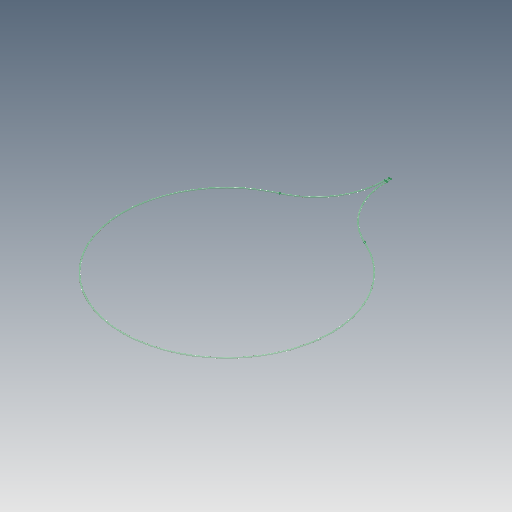
# Autodesk Inventor part: Fiber Loop
Saved by Autodesk Inventor 2020 (Build 240168000, 168)
## iProperties
Created: 2015-08-17
Part Number: Fiber Loop
Material: Glass
Document SubType Name: Modeling
Designer: Cosmic
Density: 2.18 g/cm^3
Appearance: Clear - Green 1
Author: Cosmic
Autodesk Inventor part; units mm, degrees
note: some values were not read from the file. Left out: dimensions or parameters whose unit could not be read.
ref_plane "YZ Plane" through (0, 0, 0) normal (1, 0, 0) x (0, 1, 0)
ref_plane "XZ Plane" through (0, 0, 0) normal (0, 1, 0) x (-1, 0, 0)
ref_plane "XY Plane" through (0, 0, 0) normal (0, 0, 1) x (1, 0, 0)
sketch "Sketch1" plane through (0, 0, 0) normal (0, 0, 1) x (1, 0, 0)
  arc A0 (30.463183, 68.534623) -> (-30.463183, 68.534623) centre (0, 0) ccw
  arc A1 (-30.528171, 68.68083) -> (-33.355077, 67.353281) centre (0, 0) ccw
  arc A2 (-37.826681, 66.079057) -> (-38.359263, 65.77132) centre (0, 0) ccw
  arc A3 (-38.420862, 65.920614) -> (-38.91605, 65.629498) centre (0, 0) ccw
  arc A4 (-1.3, 115.412304) -> (-101.3, 115.412304) centre (-51.3, 115.412304) ccw
  arc A5 (-1.14, 115.412304) -> (-101.46, 115.412304) centre (-51.3, 115.412304) ccw
  arc A6 (-30.528171, 68.68083) -> (-23.706504, 72.355382) centre (-51.3, 115.412304) ccw
  arc A7 (-33.355077, 67.353281) -> (-30.463183, 68.534623) centre (-51.3, 115.412304) ccw
  arc A8 (30.991211, 69.722556) -> (101.3, 115.412304) centre (51.3, 115.412304) ccw
  arc A9 (28.122774, 70.92813) -> (30.926223, 69.576349) centre (51.3, 115.412304) ccw
  arc A10 (23.190762, 72.690292) -> (23.706504, 72.355382) centre (51.3, 115.412304) ccw
  arc A11 (22.642863, 72.862822) -> (23.121211, 72.544532) centre (51.3, 115.412304) ccw
  line L0 (-51.3, 115.412304) -> (51.3, 115.412304)
  arc A12 (-33.808111, 68.401035) -> (-38.420862, 65.920614) centre (0, 0) ccw
  arc A13 (-30.926223, 69.576349) -> (-37.826681, 66.079057) centre (0, 0) ccw
  arc A14 (-37.826681, 66.079057) -> (-30.528171, 68.68083) centre (-51.3, 115.412304) ccw
  arc A15 (-38.359263, 65.77132) -> (-33.355077, 67.353281) centre (-51.3, 115.412304) ccw
  arc A16 (-38.420862, 65.920614) -> (-37.826681, 66.079057) centre (-51.3, 115.412304) ccw
  arc A17 (-38.359263, 65.77132) -> (38.359263, 65.77132) centre (0, 0) ccw
  arc A18 (-0.16, 115.412304) -> (-102.44, 115.412304) centre (-51.3, 115.412304) ccw
  arc A19 (-38.91605, 65.629498) -> (38.91605, 65.629498) centre (0, 0) ccw
  arc A20 (38.359263, 65.77132) -> (37.826681, 66.079057) centre (0, 0) ccw
  arc A21 (38.91605, 65.629498) -> (38.420862, 65.920614) centre (0, 0) ccw
  arc A22 (-102.44, 115.412304) -> (-38.420862, 65.920614) centre (-51.3, 115.412304) ccw
  arc A23 (-38.91605, 65.629498) -> (-38.359263, 65.77132) centre (-51.3, 115.412304) ccw
  arc A24 (0, 115.412304) -> (-102.6, 115.412304) centre (-51.3, 115.412304) ccw
  arc A25 (-23.706504, 72.355382) -> (-23.190762, 72.690292) centre (-51.3, 115.412304) ccw
  arc A26 (-23.190762, 72.690292) -> (-28.122774, 70.92813) centre (0, 0) ccw
  arc A27 (-23.190762, 72.690292) -> (-0.16, 115.412304) centre (-51.3, 115.412304) ccw
  arc A28 (-30.991211, 69.722556) -> (-1.3, 115.412304) centre (-51.3, 115.412304) ccw
  arc A29 (-28.122774, 70.92813) -> (-1.14, 115.412304) centre (-51.3, 115.412304) ccw
  arc A30 (-22.642863, 72.862822) -> (0, 115.412304) centre (-51.3, 115.412304) ccw
  arc A31 (-27.648555, 69.889792) -> (-30.528171, 68.68083) centre (0, 0) ccw
  arc A32 (-30.463183, 68.534623) -> (30.463183, 68.534623) centre (0, 0) ccw
  arc A33 (-33.808111, 68.401035) -> (-30.926223, 69.576349) centre (-51.3, 115.412304) ccw
  arc A34 (-101.46, 115.412304) -> (-33.808111, 68.401035) centre (-51.3, 115.412304) ccw
  arc A35 (-33.355077, 67.353281) -> (33.355077, 67.353281) centre (0, 0) ccw
  arc A36 (-101.3, 115.412304) -> (-30.991211, 69.722556) centre (-51.3, 115.412304) ccw
  arc A37 (-102.6, 115.412304) -> (-38.91605, 65.629498) centre (-51.3, 115.412304) ccw
  arc A38 (33.355077, 67.353281) -> (30.528171, 68.68083) centre (0, 0) ccw
  arc A39 (-30.991211, 69.722556) -> (-33.808111, 68.401035) centre (0, 0) ccw
  arc A40 (-30.926223, 69.576349) -> (-28.122774, 70.92813) centre (-51.3, 115.412304) ccw
  arc A41 (-30.463183, 68.534623) -> (-27.648555, 69.889792) centre (-51.3, 115.412304) ccw
  arc A42 (-27.648555, 69.889792) -> (-23.121211, 72.544532) centre (-51.3, 115.412304) ccw
  arc A43 (-28.122774, 70.92813) -> (-30.991211, 69.722556) centre (0, 0) ccw
  arc A44 (-23.706504, 72.355382) -> (-30.926223, 69.576349) centre (0, 0) ccw
  arc A45 (27.648555, 69.889792) -> (-27.648555, 69.889792) centre (0, 0) ccw
  arc A46 (-23.121211, 72.544532) -> (-22.642863, 72.862822) centre (-51.3, 115.412304) ccw
  arc A47 (-22.642863, 72.862822) -> (-23.190762, 72.690292) centre (0, 0) ccw
  arc A48 (22.642863, 72.862822) -> (-22.642863, 72.862822) centre (0, 0) ccw
  arc A49 (-23.121211, 72.544532) -> (-23.706504, 72.355382) centre (0, 0) ccw
  arc A50 (23.121211, 72.544532) -> (-23.121211, 72.544532) centre (0, 0) ccw
  arc A51 (1.14, 115.412304) -> (28.122774, 70.92813) centre (51.3, 115.412304) ccw
  arc A52 (1.3, 115.412304) -> (30.991211, 69.722556) centre (51.3, 115.412304) ccw
  arc A53 (0, 115.412304) -> (22.642863, 72.862822) centre (51.3, 115.412304) ccw
  arc A54 (0.16, 115.412304) -> (23.190762, 72.690292) centre (51.3, 115.412304) ccw
  arc A55 (23.121211, 72.544532) -> (27.648555, 69.889792) centre (51.3, 115.412304) ccw
  arc A56 (23.190762, 72.690292) -> (22.642863, 72.862822) centre (0, 0) ccw
  arc A57 (23.706504, 72.355382) -> (30.528171, 68.68083) centre (51.3, 115.412304) ccw
  arc A58 (27.648555, 69.889792) -> (30.463183, 68.534623) centre (51.3, 115.412304) ccw
  arc A59 (28.122774, 70.92813) -> (23.190762, 72.690292) centre (0, 0) ccw
  arc A60 (30.528171, 68.68083) -> (37.826681, 66.079057) centre (51.3, 115.412304) ccw
  arc A61 (23.706504, 72.355382) -> (23.121211, 72.544532) centre (0, 0) ccw
  arc A62 (30.926223, 69.576349) -> (23.706504, 72.355382) centre (0, 0) ccw
  arc A63 (30.926223, 69.576349) -> (33.808111, 68.401035) centre (51.3, 115.412304) ccw
  arc A64 (30.991211, 69.722556) -> (28.122774, 70.92813) centre (0, 0) ccw
  arc A65 (30.463183, 68.534623) -> (33.355077, 67.353281) centre (51.3, 115.412304) ccw
  arc A66 (30.528171, 68.68083) -> (27.648555, 69.889792) centre (0, 0) ccw
  arc A67 (33.355077, 67.353281) -> (38.359263, 65.77132) centre (51.3, 115.412304) ccw
  arc A68 (37.826681, 66.079057) -> (38.420862, 65.920614) centre (51.3, 115.412304) ccw
  arc A69 (101.3, 115.412304) -> (1.3, 115.412304) centre (51.3, 115.412304) ccw
  arc A70 (33.808111, 68.401035) -> (101.46, 115.412304) centre (51.3, 115.412304) ccw
  arc A71 (37.826681, 66.079057) -> (30.926223, 69.576349) centre (0, 0) ccw
  arc A72 (33.808111, 68.401035) -> (30.991211, 69.722556) centre (0, 0) ccw
  arc A73 (38.420862, 65.920614) -> (33.808111, 68.401035) centre (0, 0) ccw
  arc A74 (101.46, 115.412304) -> (1.14, 115.412304) centre (51.3, 115.412304) ccw
  arc A75 (38.359263, 65.77132) -> (38.91605, 65.629498) centre (51.3, 115.412304) ccw
  arc A76 (38.91605, 65.629498) -> (102.6, 115.412304) centre (51.3, 115.412304) ccw
  arc A77 (38.420862, 65.920614) -> (102.44, 115.412304) centre (51.3, 115.412304) ccw
  arc A78 (102.44, 115.412304) -> (0.16, 115.412304) centre (51.3, 115.412304) ccw
  arc A79 (102.6, 115.412304) -> (0, 115.412304) centre (51.3, 115.412304) ccw
  dimension "d16" = 0.16
  dimension "d17" = 0.98
  dimension "d18" = 0.16
  dimension "d19" = 150
  dimension "d20" = 0.16
  dimension "d21" = 0.98
  dimension "d22" = 0.16
  dimension "d23" = 100
  dimension "d28" = 0.16
  dimension "d29" = 0.98
  dimension "d30" = 0.16
  dimension "d31" = 100
  constraints: 181 point on circle, 80 centre point, 10 coincident, 3 tangent, 19 other
  measures "d16" radial gap between concentric circles of A1 A0
  measures "d17" radial gap between concentric circles of A2 A1
  measures "d18" radial gap between concentric circles of A3 A2
  measures "d19" diameter of A0
  measures "d20" radial gap between concentric circles of A5 A4
  measures "d21" radial gap between concentric circles of A6 A5
  measures "d22" radial gap between concentric circles of A7 A6
  measures "d23" diameter of A4
  measures "d28" radial gap between concentric circles of A9 A8
  measures "d29" radial gap between concentric circles of A10 A9
  measures "d30" radial gap between concentric circles of A11 A10
  measures "d31" diameter of A8
sketch "Sketch1 outline for Extrusion1" plane through (0, 0, 0) normal (0, 0, 1) x (1, 0, 0)
  arc A0 (-30.926223, 69.576349) -> (30.926223, 69.576349) centre (0, 0) ccw
  arc A1 (30.926223, 69.576349) -> (1.14, 115.412304) centre (51.3, 115.412304) cw
  line L0 (1.14, 115.412304) -> (0.16, 115.412304)
  arc A2 (0.16, 115.412304) -> (30.528171, 68.68083) centre (51.3, 115.412304) ccw
  arc A3 (30.528171, 68.68083) -> (-30.528171, 68.68083) centre (0, 0) cw
  arc A4 (-30.528171, 68.68083) -> (-0.16, 115.412304) centre (-51.3, 115.412304) ccw
  line L1 (-0.16, 115.412304) -> (-1.14, 115.412304)
  arc A5 (-1.14, 115.412304) -> (-30.926223, 69.576349) centre (-51.3, 115.412304) cw
extrude "Extrusion1" add sketch "Sketch1 outline for Extrusion1" along normal mid plane 0.98
fillet "Fillet1" radius 0.49 11 edges at (0, -75.16, 0.49) (8.4189, 87.5463, 0.49) (-8.4189, 87.5463, 0.49) (0, -76.14, 0.49) (9.2407, 88.0803, 0.49) (-9.2407, 88.0803, 0.49) (0, -76.14, -0.49) (-9.2407, 88.0803, -0.49) (9.2407, 88.0803, -0.49) (0, -75.16, -0.49) (8.4189, 87.5463, -0.49)
sketch "Sketch2" plane through (0.65, 115.412304, 0) normal (0, 1, 0) x (1, 0, 0)
  circle A0 centre (0, 0) radius 0.49 projected
  circle A1 centre (-1.3, 0) radius 0.49 projected
  point P0 (-0.65, 0)
extrude "Extrusion2" add sketch "Sketch2" along normal blind 3
equation "\"d16\" = OpticalFiberClearence + 0.01 * OpticalFiberDiameter"
equation "\"d17\" = 0.98 * OpticalFiberDiameter"
equation "\"d18\" = OpticalFiberClearence + 0.01 * OpticalFiberDiameter"
equation "\"d20\" = OpticalFiberClearence + 0.01 * OpticalFiberDiameter"
equation "\"d21\" = 0.98 * OpticalFiberDiameter"
equation "\"d22\" = OpticalFiberClearence + 0.01 * OpticalFiberDiameter"
equation "\"d23\" = LoopSmallTrackDiameter"
equation "\"d28\" = OpticalFiberClearence + 0.01 * OpticalFiberDiameter"
equation "\"d29\" = 0.98 * OpticalFiberDiameter"
equation "\"d30\" = OpticalFiberClearence + 0.01 * OpticalFiberDiameter"
equation "\"d31\" = LoopSmallTrackDiameter"
equation "\"d36\" = 0.98 * OpticalFiberDiameter"
equation "\"d38\" = 0.49 * OpticalFiberDiameter"
equation "\"d39\" = ScintillatorEdgeClearence"
equation "\"OpticalFiberDiameter\" = 1"
equation "\"OpticalFiberClearence\" = 0.15"
equation "\"ScintillatorEdgeClearence\" = 3"
equation "\"MPPCDepth\" = 1"
equation "\"LoopLargeTrackRatio\" = 1.5"
equation "\"LoopSmallTrackDiameter\" = 100"
equation "\"d24\" = 0.05"
equation "\"d25\" = 1"
equation "\"d32\" = 0.05"
equation "\"d33\" = 1"
equation "\"FiberSensorClerence\" = 0.5"
equation "\"SmallTrackDiameter\" = 175"
equation "\"ShallowTrackDepth\" = 1.3"
equation "\"MPPCClearence\" = 0.075"
equation "\"MPPCSensorClearence\" = 1.45"
equation "\"MPPCSensorOffsett\" = 2.105"
equation "\"MPPCWidth\" = 5.9"
equation "\"MPPCHeight\" = 6.55"
equation "\"FiberEdgeOffsett\" = 5"
equation "\"LongFiberAngle\" = 30deg"
equation "\"ShortFiberAngle\" = 78deg"
equation "\"MountingScrewDepth\" = 4"
equation "\"cornerChamfer\" = 25.4"
equation "\"mountingSpacing\" = 18"
equation "\"silveringThickness\" = 0.2"
body "Solid1"
